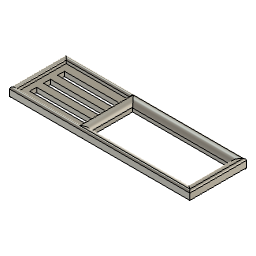
plastic_rack (Autodesk Fusion 360 design; units mm, degrees)
Autodesk Fusion 360 part; units mm, degrees
sketch "Sketch1" plane through (0, 0, 0) normal (0, 0, 1) x (1, 0, 0)
  line L0 (0, 0) -> (150, 0)
  line L1 (150, 0) -> (150, 43)
  line L2 (150, 43) -> (0, 43)
  line L3 (0, 43) -> (0, 0)
  line L4 (0, 43) -> (5, 43)
  line L5 (5, 43) -> (5, 0)
  line L6 (5, 0) -> (0, 0)
  line L7 (0, 0) -> (0, 43)
  line L8 (5, 0) -> (55, 0)
  line L9 (55, 0) -> (55, 6.5)
  line L10 (55, 6.5) -> (5, 6.5)
  line L11 (5, 6.5) -> (5, 0)
  line L12 (5, 6.5) -> (55, 6.5)
  line L13 (55, 6.5) -> (55, 12.5)
  line L14 (55, 12.5) -> (5, 12.5)
  line L15 (5, 12.5) -> (5, 6.5)
  line L16 (5, 12.5) -> (55, 12.5)
  line L17 (55, 12.5) -> (55, 18.5)
  line L18 (55, 18.5) -> (5, 18.5)
  line L19 (5, 18.5) -> (5, 12.5)
  line L20 (5, 18.5) -> (55, 18.5)
  line L21 (55, 18.5) -> (55, 24.5)
  line L22 (55, 24.5) -> (5, 24.5)
  line L23 (5, 24.5) -> (5, 18.5)
  line L24 (5, 24.5) -> (55, 24.5)
  line L25 (55, 24.5) -> (55, 30.5)
  line L26 (55, 30.5) -> (5, 30.5)
  line L27 (5, 30.5) -> (5, 24.5)
  line L28 (5, 30.5) -> (55, 30.5)
  line L29 (55, 30.5) -> (55, 36.5)
  line L30 (55, 36.5) -> (5, 36.5)
  line L31 (5, 36.5) -> (5, 30.5)
  line L32 (5, 43) -> (55, 43)
  line L33 (55, 43) -> (55, 36.5)
  line L34 (55, 36.5) -> (5, 36.5)
  line L35 (5, 36.5) -> (5, 43)
  line L36 (150, 0) -> (144, 0)
  line L37 (144, 0) -> (144, 3.5)
  line L38 (144, 3.5) -> (150, 3.5)
  line L39 (150, 3.5) -> (150, 0)
  line L40 (55, 43) -> (61, 43)
  line L41 (61, 43) -> (61, 39.5)
  line L42 (61, 39.5) -> (55, 39.5)
  line L43 (55, 39.5) -> (55, 43)
  line L44 (61, 39.5) -> (144, 39.5)
  line L45 (144, 39.5) -> (144, 3.5)
  line L46 (144, 3.5) -> (61, 3.5)
  line L47 (61, 3.5) -> (61, 39.5)
  line L48 (0, 0) -> (-3, 0)
  line L49 (-3, 0) -> (-3, -3)
  line L50 (-3, -3) -> (0, -3)
  line L51 (0, -3) -> (0, 0)
  line L52 (-3, -3) -> (153, -3)
  line L53 (153, -3) -> (153, 46)
  line L54 (153, 46) -> (-3, 46)
  line L55 (-3, 46) -> (-3, -3)
  dimension "d1" = 150
  dimension "d2" = 43
  dimension "d3" = 50
  dimension "d4" = 6.5
  dimension "d5" = 50
  dimension "d6" = 6
  dimension "d7" = 50
  dimension "d8" = 6
  dimension "d9" = 50
  dimension "d10" = 6
  dimension "d11" = 50
  dimension "d12" = 6
  dimension "d13" = 50
  dimension "d14" = 6
  dimension "d17" = 6
  dimension "d18" = 3.5
  dimension "d19" = 6
  dimension "d20" = 3.5
  dimension "d25" = 3
  dimension "d26" = 3
  dimension "d27" = 156
  dimension "d28" = 49
  constraint horizontal L0
  constraint vertical L1
  constraint horizontal L2
  constraint vertical L3
  constraint coincident L0.start L3.end
  constraint horizontal L4
  constraint vertical L5
  constraint horizontal L6
  constraint vertical L7
  constraint coincident L0 L5.end
  constraint horizontal L8
  constraint vertical L9
  constraint horizontal L10
  constraint vertical L11
  constraint horizontal L12
  constraint vertical L13
  constraint horizontal L14
  constraint vertical L15
  constraint horizontal L16
  constraint vertical L17
  constraint horizontal L18
  constraint vertical L19
  constraint horizontal L20
  constraint vertical L21
  constraint horizontal L22
  constraint vertical L23
  constraint horizontal L24
  constraint vertical L25
  constraint horizontal L26
  constraint vertical L27
  constraint horizontal L28
  constraint vertical L29
  constraint horizontal L30
  constraint vertical L31
  constraint horizontal L32
  constraint vertical L33
  constraint horizontal L34
  constraint vertical L35
  constraint horizontal L36
  constraint vertical L37
  constraint horizontal L38
  constraint vertical L39
  constraint horizontal L40
  constraint vertical L41
  constraint horizontal L42
  constraint vertical L43
  constraint horizontal L44
  constraint vertical L45
  constraint horizontal L46
  constraint vertical L47
  constraint horizontal L48
  constraint vertical L49
  constraint horizontal L50
  constraint vertical L51
  constraint horizontal L52
  constraint vertical L53
  constraint horizontal L54
  constraint vertical L55
  measures "d1" distance of L0.start L0.end
  measures "d2" distance of L0.start L2.end
  measures "d3" distance of L5.end L8.end
  measures "d4" distance of L5.end L10.end
  measures "d5" distance of L10.end L9.end
  measures "d6" distance of L10.end L14.end
  measures "d7" distance of L14.end L13.end
  measures "d8" distance of L14.end L18.end
  measures "d9" distance of L18.end L17.end
  measures "d10" distance of L18.end L22.end
  measures "d11" distance of L22.end L21.end
  measures "d12" distance of L22.end L26.end
  measures "d13" distance of L26.end L25.end
  measures "d14" distance of L26.end L30.end
  measures "d17" distance of L0.end L36.end
  measures "d18" distance of L0.end L38.end
  measures "d19" distance of L32.end L40.end
  measures "d20" distance of L32.end L42.end
  measures "d25" distance of L0.start L48.end
  measures "d26" distance of L0.start L50.end
  measures "d27" distance of L49.end L52.end
  measures "d28" distance of L49.end L54.end
extrude "Extrude2" add sketch "Sketch1" along normal blind 4 contours L0 L2 L3 L4 L5 L6 L7 L11 L15 L19 L23 L27 L31 L35 | L0 L5 L8 L9 L10 L11 L12 | L2 L5 L30 L32 L33 L34 L35 L43 | L5 L14 L16 L17 L18 L19 L20 | L5 L22 L24 L25 L26 L27 L28
extrude "Extrude3" add sketch "Sketch1" along normal blind 8 contours L0 L9 L13 L17 L21 L25 L29 L33 L37 L42 L46 L47 | L0 L1 L36 L37 L38 L39 | L2 L33 L40 L41 L42 L43 | L1 L2 L38 L41 L44 L45
extrude "Extrude4" add sketch "Sketch1" along normal blind 8
fillet "Fillet1" radius 1.5 4 edges at (55, 21.5, 8) (27.5, 43, 8) (0, 21.5, 8) (27.5, 0, 8)
fillet "Fillet2" radius 1.5 4 edges at (75, -3, 8) (-3, 21.5, 8) (75, 46, 8) (153, 21.5, 8)
fillet "Fillet3" radius 4.5 1 edges at (61, 21.5, 8)
fillet "Fillet4" radius 5 2 edges at (100.25, 3.5, 8) (100.25, 39.5, 8)
fillet "Fillet5" radius 7.5 1 edges at (144, 21.5, 8)
fillet "Fillet6" radius 1 4 edges at (75, -3, 0) (-3, 21.5, 0) (75, 46, 0) (153, 21.5, 0)
